Autodesk Fusion 360 part; units mm, degrees
(part 2 of 3)
sketch "Skizze15" plane through (0, 0, -33) normal (0, 0, -1) x (1, 0, 0)
  line L0 (-5.3, -15.5) -> (-3.8, -15.5)
  line L1 (-3.8, -15.5) -> (-3.8, -12.5)
  line L2 (-3.8, -12.5) -> (-2, -12.5)
  line L3 (-2, -12.5) -> (-2, -15.5)
  line L4 (-2, -15.5) -> (-0.5, -15.5)
  line L5 (-0.5, -15.5) -> (-0.5, 0.5)
  line L6 (-0.5, 0.5) -> (77.5, 0.5)
  line L7 (77.5, 0.5) -> (77.5, -50)
  line L8 (77.5, -50) -> (-0.5, -50)
  line L9 (-0.5, -50) -> (-0.5, -21.5)
  line L10 (-0.5, -21.5) -> (-2, -21.5)
  line L11 (-2, -21.5) -> (-2, -24.5)
  line L12 (-2, -24.5) -> (-3.8, -24.5)
  line L13 (-3.8, -24.5) -> (-3.8, -21.5)
  line L14 (-3.8, -21.5) -> (-5.3, -21.5)
  line L15 (-5.3, -21.5) -> (-5.3, -26)
  line L16 (-5.3, -26) -> (-2, -26)
  line L17 (-2, -26) -> (-2, -51.5)
  line L18 (-2, -51.5) -> (79, -51.5)
  line L19 (79, -51.5) -> (79, 2)
  line L20 (79, 2) -> (-2, 2)
  line L21 (-2, 2) -> (-2, -11)
  line L22 (-2, -11) -> (-5.3, -11)
  line L23 (-5.3, -11) -> (-5.3, -15.5)
  line L24 (-0.4, -21.4) -> (-2.1, -21.4)
  line L25 (-2.1, -21.4) -> (-2.1, -24.4)
  line L26 (-2.1, -24.4) -> (-3.7, -24.4)
  line L27 (-3.7, -24.4) -> (-3.7, -21.4)
  line L28 (-3.7, -21.4) -> (-5.4, -21.4)
  line L29 (-5.4, -21.4) -> (-5.4, -26.1)
  line L30 (-5.4, -26.1) -> (-2.1, -26.1)
  line L31 (-2.1, -26.1) -> (-2.1, -51.6)
  line L32 (-2.1, -51.6) -> (79.1, -51.6)
  line L33 (79.1, -51.6) -> (79.1, 2.1)
  line L34 (79.1, 2.1) -> (-2.1, 2.1)
  line L35 (-2.1, 2.1) -> (-2.1, -10.9)
  line L36 (-2.1, -10.9) -> (-5.4, -10.9)
  line L37 (-5.4, -10.9) -> (-5.4, -15.6)
  line L38 (-5.4, -15.6) -> (-3.7, -15.6)
  line L39 (-3.7, -15.6) -> (-3.7, -12.6)
  line L40 (-3.7, -12.6) -> (-2.1, -12.6)
  line L41 (-2.1, -12.6) -> (-2.1, -15.6)
  line L42 (-2.1, -15.6) -> (-0.4, -15.6)
  line L43 (-0.4, -15.6) -> (-0.4, 0.4)
  line L44 (-0.4, 0.4) -> (77.4, 0.4)
  line L45 (77.4, 0.4) -> (77.4, -49.9)
  line L46 (77.4, -49.9) -> (-0.4, -49.9)
  line L47 (-0.4, -49.9) -> (-0.4, -21.4)
  line L48 (-0.4, -21.4) -> (-0.4, -15.6)
  line L49 (-0.4, -49.9) -> (77.4, -49.9)
  line L50 (77.4, -49.9) -> (77.4, 0.4)
  line L51 (77.4, 0.4) -> (-0.4, 0.4)
  line L52 (-0.4, 0.4) -> (-0.4, -49.9)
  line L53 (75.9, -1.1) -> (1.1, -1.1)
  line L54 (1.1, -1.1) -> (1.1, -48.4)
  line L55 (1.1, -48.4) -> (75.9, -48.4)
  line L56 (75.9, -48.4) -> (75.9, -1.1)
  line L57 (-5.4, -21.4) -> (-5.4, -15.5)
  line L58 (-5.3, -21.5) -> (-5.3, -15.5)
  dimension "d73" = 0.1
  dimension "d74" = -1.5
  constraint horizontal L49
  constraint vertical L50
  constraint horizontal L51
  constraint vertical L52
  constraint coincident L37 L57.end
  constraint coincident L14.end L15.start
  constraint coincident L0.start L23.end
extrude "Extrusion20" add sketch "Skizze15" along normal blind 1.5 separate body contours L0 L1 L2 L3 L4 L5 L6 L7 L8 L9 L10 L11 L12 L13 L14 L15 L16 L17 L18 L19 L20 L21 L22 L23 | L0 L1 L2 L3 L4 L5 L6 L7 L8 L9 L10 L11 L12 L13 L14 L24 L25 L26 L27 L28 L38 L39 L40 L41 L42 L43 L44 L45 L46 L47 L49 L50 L51 L52 L58 | L24 L25 L26 L27 L28 L38 L39 L40 L41 L42 L48 L52 L58 | L43 L44 L45 L46 L47 L48 L49 L50 L51 L52 | L53 L54 L55 L56 makes body 4
sketch "Skizze16" plane through (0, 0, -34.5) normal (0, 0, -1) x (1, 0, 0)
  line L0 (-5.3, -26) -> (-2, -26)
  line L1 (-2, -26) -> (-2, -51.5)
  line L2 (-2, -51.5) -> (79, -51.5)
  line L3 (79, -51.5) -> (79, 2)
  line L4 (79, 2) -> (-2, 2)
  line L5 (-2, 2) -> (-2, -11)
  line L6 (-2, -11) -> (-5.3, -11)
  line L7 (-5.3, -11) -> (-5.3, -26)
  line L8 (1.1, -48.4) -> (75.9, -48.4)
  line L9 (75.9, -48.4) -> (75.9, -1.1)
  line L10 (75.9, -1.1) -> (1.1, -1.1)
  line L11 (1.1, -1.1) -> (1.1, -48.4)
  line L12 (1.1, -48.4) -> (75.9, -48.4)
  line L13 (-0.4, -49.9) -> (-0.4, 0.4)
  line L14 (-0.4, 0.4) -> (77.4, 0.4)
  line L15 (77.4, 0.4) -> (77.4, -49.9)
  line L16 (77.4, -49.9) -> (-0.4, -49.9)
  line L17 (-2, -51.5) -> (79, 2) construction
  line L18 (-2, 2) -> (79, -51.5) construction
  line L19 (53, -5.5) -> (24, -5.5)
  arc A0 (24, -5.5) -> (24, -44) centre (24, -24.75) ccw
  line L20 (24, -44) -> (53, -44)
  arc A1 (53, -44) -> (53, -5.5) centre (53, -24.75) ccw
  line L21 (53, -24.75) -> (24, -24.75) construction
  line L22 (-89.8785, -69.1132) -> (-94.8785, -66.2265)
  line L23 (-94.8785, -66.2265) -> (-99.8785, -69.1132)
  line L24 (-99.8785, -69.1132) -> (-99.8785, -74.8868)
  line L25 (-99.8785, -74.8868) -> (-94.8785, -77.7735)
  line L26 (-94.8785, -77.7735) -> (-89.8785, -74.8868)
  line L27 (-89.8785, -74.8868) -> (-89.8785, -69.1132)
  line L28 (-94.8785, -77.7735) -> (6, -77.7735)
  line L29 (-83.1871, -71.0235) -> (-78.1871, -68.1368)
  line L30 (-78.1871, -68.1368) -> (-78.1871, -62.3632)
  line L31 (-78.1871, -62.3632) -> (-83.1871, -59.4765)
  line L32 (-83.1871, -59.4765) -> (-88.1871, -62.3632)
  line L33 (-88.1871, -62.3632) -> (-88.1871, -68.1368)
  line L34 (-88.1871, -68.1368) -> (-83.1871, -71.0235)
  line L35 (-71.4958, -64.2735) -> (-66.4958, -61.3868)
  line L36 (-66.4958, -61.3868) -> (-66.4958, -55.6132)
  line L37 (-66.4958, -55.6132) -> (-71.4958, -52.7265)
  line L38 (-71.4958, -52.7265) -> (-76.4958, -55.6132)
  line L39 (-76.4958, -55.6132) -> (-76.4958, -61.3868)
  line L40 (-76.4958, -61.3868) -> (-71.4958, -64.2735)
  line L41 (-59.8044, -57.5235) -> (-54.8044, -54.6368)
  line L42 (-54.8044, -54.6368) -> (-54.8044, -48.8632)
  line L43 (-54.8044, -48.8632) -> (-59.8044, -45.9765)
  line L44 (-59.8044, -45.9765) -> (-64.8044, -48.8632)
  line L45 (-64.8044, -48.8632) -> (-64.8044, -54.6368)
  line L46 (-64.8044, -54.6368) -> (-59.8044, -57.5235)
  line L47 (-48.1131, -50.7735) -> (-43.1131, -47.8868)
  line L48 (-43.1131, -47.8868) -> (-43.1131, -42.1132)
  line L49 (-43.1131, -42.1132) -> (-48.1131, -39.2265)
  line L50 (-48.1131, -39.2265) -> (-53.1131, -42.1132)
  line L51 (-53.1131, -42.1132) -> (-53.1131, -47.8868)
  line L52 (-53.1131, -47.8868) -> (-48.1131, -50.7735)
  line L53 (-36.4217, -44.0235) -> (-31.4217, -41.1368)
  line L54 (-31.4217, -41.1368) -> (-31.4217, -35.3632)
  line L55 (-31.4217, -35.3632) -> (-36.4217, -32.4765)
  line L56 (-36.4217, -32.4765) -> (-41.4217, -35.3632)
  line L57 (-41.4217, -35.3632) -> (-41.4217, -41.1368)
  line L58 (-41.4217, -41.1368) -> (-36.4217, -44.0235)
  line L59 (-24.7304, -37.2735) -> (-19.7304, -34.3868)
  line L60 (-19.7304, -34.3868) -> (-19.7304, -28.6132)
  line L61 (-19.7304, -28.6132) -> (-24.7304, -25.7265)
  line L62 (-24.7304, -25.7265) -> (-29.7304, -28.6132)
  line L63 (-29.7304, -28.6132) -> (-29.7304, -34.3868)
  line L64 (-29.7304, -34.3868) -> (-24.7304, -37.2735)
  line L65 (-13.0391, -30.5235) -> (-8.0391, -27.6368)
  line L66 (-8.0391, -27.6368) -> (-8.0391, -21.8632)
  line L67 (-8.0391, -21.8632) -> (-13.0391, -18.9765)
  line L68 (-13.0391, -18.9765) -> (-18.0391, -21.8632)
  line L69 (-18.0391, -21.8632) -> (-18.0391, -27.6368)
  line L70 (-18.0391, -27.6368) -> (-13.0391, -30.5235)
  line L71 (-1.3477, -23.7735) -> (3.6523, -20.8868)
  line L72 (3.6523, -20.8868) -> (3.6523, -15.1132)
  line L73 (3.6523, -15.1132) -> (-1.3477, -12.2265)
  line L74 (-1.3477, -12.2265) -> (-6.3477, -15.1132)
  line L75 (-6.3477, -15.1132) -> (-6.3477, -20.8868)
  line L76 (-6.3477, -20.8868) -> (-1.3477, -23.7735)
  line L77 (10.3436, -17.0235) -> (15.3436, -14.1368)
  line L78 (15.3436, -14.1368) -> (15.3436, -8.3632)
  line L79 (15.3436, -8.3632) -> (10.3436, -5.4765)
  line L80 (10.3436, -5.4765) -> (5.3436, -8.3632)
  line L81 (5.3436, -8.3632) -> (5.3436, -14.1368)
  line L82 (5.3436, -14.1368) -> (10.3436, -17.0235)
  line L83 (22.035, -10.2735) -> (27.035, -7.3868)
  line L84 (27.035, -7.3868) -> (27.035, -1.6132)
  line L85 (27.035, -1.6132) -> (22.035, 1.2735)
  line L86 (22.035, 1.2735) -> (17.035, -1.6132)
  line L87 (17.035, -1.6132) -> (17.035, -7.3868)
  line L88 (17.035, -7.3868) -> (22.035, -10.2735)
  line L89 (-70.8785, -77.7735) -> (-65.8785, -74.8868)
  line L90 (-65.8785, -74.8868) -> (-65.8785, -69.1132)
  line L91 (-65.8785, -69.1132) -> (-70.8785, -66.2265)
  line L92 (-70.8785, -66.2265) -> (-75.8785, -69.1132)
  line L93 (-75.8785, -69.1132) -> (-75.8785, -74.8868)
  line L94 (-75.8785, -74.8868) -> (-70.8785, -77.7735)
  line L95 (-59.1871, -71.0235) -> (-54.1871, -68.1368)
  line L96 (-54.1871, -68.1368) -> (-54.1871, -62.3632)
  line L97 (-54.1871, -62.3632) -> (-59.1871, -59.4765)
  line L98 (-59.1871, -59.4765) -> (-64.1871, -62.3632)
  line L99 (-64.1871, -62.3632) -> (-64.1871, -68.1368)
  line L100 (-64.1871, -68.1368) -> (-59.1871, -71.0235)
  line L101 (-47.4958, -64.2735) -> (-42.4958, -61.3868)
  line L102 (-42.4958, -61.3868) -> (-42.4958, -55.6132)
  line L103 (-42.4958, -55.6132) -> (-47.4958, -52.7265)
  line L104 (-47.4958, -52.7265) -> (-52.4958, -55.6132)
  line L105 (-52.4958, -55.6132) -> (-52.4958, -61.3868)
  line L106 (-52.4958, -61.3868) -> (-47.4958, -64.2735)
  line L107 (-35.8044, -57.5235) -> (-30.8044, -54.6368)
  line L108 (-30.8044, -54.6368) -> (-30.8044, -48.8632)
  line L109 (-30.8044, -48.8632) -> (-35.8044, -45.9765)
  line L110 (-35.8044, -45.9765) -> (-40.8044, -48.8632)
  line L111 (-40.8044, -48.8632) -> (-40.8044, -54.6368)
  line L112 (-40.8044, -54.6368) -> (-35.8044, -57.5235)
  line L113 (-24.1131, -50.7735) -> (-19.1131, -47.8868)
  line L114 (-19.1131, -47.8868) -> (-19.1131, -42.1132)
  line L115 (-19.1131, -42.1132) -> (-24.1131, -39.2265)
  line L116 (-24.1131, -39.2265) -> (-29.1131, -42.1132)
  line L117 (-29.1131, -42.1132) -> (-29.1131, -47.8868)
  line L118 (-29.1131, -47.8868) -> (-24.1131, -50.7735)
  line L119 (-12.4217, -44.0235) -> (-7.4217, -41.1368)
  line L120 (-7.4217, -41.1368) -> (-7.4217, -35.3632)
  line L121 (-7.4217, -35.3632) -> (-12.4217, -32.4765)
  line L122 (-12.4217, -32.4765) -> (-17.4217, -35.3632)
  line L123 (-17.4217, -35.3632) -> (-17.4217, -41.1368)
  line L124 (-17.4217, -41.1368) -> (-12.4217, -44.0235)
  line L125 (-0.7304, -37.2735) -> (4.2696, -34.3868)
  line L126 (4.2696, -34.3868) -> (4.2696, -28.6132)
  line L127 (4.2696, -28.6132) -> (-0.7304, -25.7265)
  line L128 (-0.7304, -25.7265) -> (-5.7304, -28.6132)
  line L129 (-5.7304, -28.6132) -> (-5.7304, -34.3868)
  line L130 (-5.7304, -34.3868) -> (-0.7304, -37.2735)
  line L131 (10.9609, -30.5235) -> (15.9609, -27.6368)
  line L132 (15.9609, -27.6368) -> (15.9609, -21.8632)
  line L133 (15.9609, -21.8632) -> (10.9609, -18.9765)
  line L134 (10.9609, -18.9765) -> (5.9609, -21.8632)
  line L135 (5.9609, -21.8632) -> (5.9609, -27.6368)
  line L136 (5.9609, -27.6368) -> (10.9609, -30.5235)
  line L137 (22.6523, -23.7735) -> (27.6523, -20.8868)
  line L138 (27.6523, -20.8868) -> (27.6523, -15.1132)
  line L139 (27.6523, -15.1132) -> (22.6523, -12.2265)
  line L140 (22.6523, -12.2265) -> (17.6523, -15.1132)
  line L141 (17.6523, -15.1132) -> (17.6523, -20.8868)
  line L142 (17.6523, -20.8868) -> (22.6523, -23.7735)
  line L143 (34.3436, -17.0235) -> (39.3436, -14.1368)
  line L144 (39.3436, -14.1368) -> (39.3436, -8.3632)
  line L145 (39.3436, -8.3632) -> (34.3436, -5.4765)
  line L146 (34.3436, -5.4765) -> (29.3436, -8.3632)
  line L147 (29.3436, -8.3632) -> (29.3436, -14.1368)
  line L148 (29.3436, -14.1368) -> (34.3436, -17.0235)
  line L149 (46.035, -10.2735) -> (51.035, -7.3868)
  line L150 (51.035, -7.3868) -> (51.035, -1.6132)
  line L151 (51.035, -1.6132) -> (46.035, 1.2735)
  line L152 (46.035, 1.2735) -> (41.035, -1.6132)
  line L153 (41.035, -1.6132) -> (41.035, -7.3868)
  line L154 (41.035, -7.3868) -> (46.035, -10.2735)
  line L155 (-46.8785, -77.7735) -> (-41.8785, -74.8868)
  line L156 (-41.8785, -74.8868) -> (-41.8785, -69.1132)
  line L157 (-41.8785, -69.1132) -> (-46.8785, -66.2265)
  line L158 (-46.8785, -66.2265) -> (-51.8785, -69.1132)
  line L159 (-51.8785, -69.1132) -> (-51.8785, -74.8868)
  line L160 (-51.8785, -74.8868) -> (-46.8785, -77.7735)
  line L161 (-35.1871, -71.0235) -> (-30.1871, -68.1368)
  line L162 (-30.1871, -68.1368) -> (-30.1871, -62.3632)
  line L163 (-30.1871, -62.3632) -> (-35.1871, -59.4765)
  line L164 (-35.1871, -59.4765) -> (-40.1871, -62.3632)
  line L165 (-40.1871, -62.3632) -> (-40.1871, -68.1368)
  line L166 (-40.1871, -68.1368) -> (-35.1871, -71.0235)
  line L167 (-23.4958, -64.2735) -> (-18.4958, -61.3868)
  line L168 (-18.4958, -61.3868) -> (-18.4958, -55.6132)
  line L169 (-18.4958, -55.6132) -> (-23.4958, -52.7265)
  line L170 (-23.4958, -52.7265) -> (-28.4958, -55.6132)
  line L171 (-28.4958, -55.6132) -> (-28.4958, -61.3868)
  line L172 (-28.4958, -61.3868) -> (-23.4958, -64.2735)
  line L173 (-11.8044, -57.5235) -> (-6.8044, -54.6368)
  line L174 (-6.8044, -54.6368) -> (-6.8044, -48.8632)
  line L175 (-6.8044, -48.8632) -> (-11.8044, -45.9765)
  line L176 (-11.8044, -45.9765) -> (-16.8044, -48.8632)
  line L177 (-16.8044, -48.8632) -> (-16.8044, -54.6368)
  line L178 (-16.8044, -54.6368) -> (-11.8044, -57.5235)
  line L179 (-0.1131, -50.7735) -> (4.8869, -47.8868)
  line L180 (4.8869, -47.8868) -> (4.8869, -42.1132)
  line L181 (4.8869, -42.1132) -> (-0.1131, -39.2265)
  line L182 (-0.1131, -39.2265) -> (-5.1131, -42.1132)
  line L183 (-5.1131, -42.1132) -> (-5.1131, -47.8868)
  line L184 (-5.1131, -47.8868) -> (-0.1131, -50.7735)
  line L185 (11.5783, -44.0235) -> (16.5783, -41.1368)
  line L186 (16.5783, -41.1368) -> (16.5783, -35.3632)
  line L187 (16.5783, -35.3632) -> (11.5783, -32.4765)
  line L188 (11.5783, -32.4765) -> (6.5783, -35.3632)
  line L189 (6.5783, -35.3632) -> (6.5783, -41.1368)
  line L190 (6.5783, -41.1368) -> (11.5783, -44.0235)
  line L191 (23.2696, -37.2735) -> (28.2696, -34.3868)
  line L192 (28.2696, -34.3868) -> (28.2696, -28.6132)
  line L193 (28.2696, -28.6132) -> (23.2696, -25.7265)
  line L194 (23.2696, -25.7265) -> (18.2696, -28.6132)
  line L195 (18.2696, -28.6132) -> (18.2696, -34.3868)
  line L196 (18.2696, -34.3868) -> (23.2696, -37.2735)
  line L197 (34.9609, -30.5235) -> (39.9609, -27.6368)
  line L198 (39.9609, -27.6368) -> (39.9609, -21.8632)
  line L199 (39.9609, -21.8632) -> (34.9609, -18.9765)
  line L200 (34.9609, -18.9765) -> (29.9609, -21.8632)
  line L201 (29.9609, -21.8632) -> (29.9609, -27.6368)
  line L202 (29.9609, -27.6368) -> (34.9609, -30.5235)
  line L203 (46.6523, -23.7735) -> (51.6523, -20.8868)
  line L204 (51.6523, -20.8868) -> (51.6523, -15.1132)
  line L205 (51.6523, -15.1132) -> (46.6523, -12.2265)
  line L206 (46.6523, -12.2265) -> (41.6523, -15.1132)
  line L207 (41.6523, -15.1132) -> (41.6523, -20.8868)
  line L208 (41.6523, -20.8868) -> (46.6523, -23.7735)
  line L209 (58.3436, -17.0235) -> (63.3436, -14.1368)
  line L210 (63.3436, -14.1368) -> (63.3436, -8.3632)
  line L211 (63.3436, -8.3632) -> (58.3436, -5.4765)
  line L212 (58.3436, -5.4765) -> (53.3436, -8.3632)
  line L213 (53.3436, -8.3632) -> (53.3436, -14.1368)
  line L214 (53.3436, -14.1368) -> (58.3436, -17.0235)
  line L215 (70.035, -10.2735) -> (75.035, -7.3868)
  line L216 (75.035, -7.3868) -> (75.035, -1.6132)
  line L217 (75.035, -1.6132) -> (70.035, 1.2735)
  line L218 (70.035, 1.2735) -> (65.035, -1.6132)
  line L219 (65.035, -1.6132) -> (65.035, -7.3868)
  line L220 (65.035, -7.3868) -> (70.035, -10.2735)
  line L221 (-22.8785, -77.7735) -> (-17.8785, -74.8868)
  line L222 (-17.8785, -74.8868) -> (-17.8785, -69.1132)
  line L223 (-17.8785, -69.1132) -> (-22.8785, -66.2265)
  line L224 (-22.8785, -66.2265) -> (-27.8785, -69.1132)
  line L225 (-27.8785, -69.1132) -> (-27.8785, -74.8868)
  line L226 (-27.8785, -74.8868) -> (-22.8785, -77.7735)
  line L227 (-11.1871, -71.0235) -> (-6.1871, -68.1368)
  line L228 (-6.1871, -68.1368) -> (-6.1871, -62.3632)
  line L229 (-6.1871, -62.3632) -> (-11.1871, -59.4765)
  line L230 (-11.1871, -59.4765) -> (-16.1871, -62.3632)
  line L231 (-16.1871, -62.3632) -> (-16.1871, -68.1368)
  line L232 (-16.1871, -68.1368) -> (-11.1871, -71.0235)
  line L233 (0.5042, -64.2735) -> (5.5042, -61.3868)
  line L234 (5.5042, -61.3868) -> (5.5042, -55.6132)
  line L235 (5.5042, -55.6132) -> (0.5042, -52.7265)
  line L236 (0.5042, -52.7265) -> (-4.4958, -55.6132)
  line L237 (-4.4958, -55.6132) -> (-4.4958, -61.3868)
  line L238 (-4.4958, -61.3868) -> (0.5042, -64.2735)
  line L239 (12.1956, -57.5235) -> (17.1956, -54.6368)
  line L240 (17.1956, -54.6368) -> (17.1956, -48.8632)
  line L241 (17.1956, -48.8632) -> (12.1956, -45.9765)
  line L242 (12.1956, -45.9765) -> (7.1956, -48.8632)
  line L243 (7.1956, -48.8632) -> (7.1956, -54.6368)
  line L244 (7.1956, -54.6368) -> (12.1956, -57.5235)
  line L245 (23.8869, -50.7735) -> (28.8869, -47.8868)
  line L246 (28.8869, -47.8868) -> (28.8869, -42.1132)
  line L247 (28.8869, -42.1132) -> (23.8869, -39.2265)
  line L248 (23.8869, -39.2265) -> (18.8869, -42.1132)
  line L249 (18.8869, -42.1132) -> (18.8869, -47.8868)
  line L250 (18.8869, -47.8868) -> (23.8869, -50.7735)
  line L251 (35.5783, -44.0235) -> (40.5783, -41.1368)
  line L252 (40.5783, -41.1368) -> (40.5783, -35.3632)
  line L253 (40.5783, -35.3632) -> (35.5783, -32.4765)
  line L254 (35.5783, -32.4765) -> (30.5783, -35.3632)
  line L255 (30.5783, -35.3632) -> (30.5783, -41.1368)
  line L256 (30.5783, -41.1368) -> (35.5783, -44.0235)
  line L257 (47.2696, -37.2735) -> (52.2696, -34.3868)
  line L258 (52.2696, -34.3868) -> (52.2696, -28.6132)
  line L259 (52.2696, -28.6132) -> (47.2696, -25.7265)
  line L260 (47.2696, -25.7265) -> (42.2696, -28.6132)
  line L261 (42.2696, -28.6132) -> (42.2696, -34.3868)
  line L262 (42.2696, -34.3868) -> (47.2696, -37.2735)
  line L263 (58.9609, -30.5235) -> (63.9609, -27.6368)
  line L264 (63.9609, -27.6368) -> (63.9609, -21.8632)
  line L265 (63.9609, -21.8632) -> (58.9609, -18.9765)
  line L266 (58.9609, -18.9765) -> (53.9609, -21.8632)
  line L267 (53.9609, -21.8632) -> (53.9609, -27.6368)
  line L268 (53.9609, -27.6368) -> (58.9609, -30.5235)
  line L269 (70.6523, -23.7735) -> (75.6523, -20.8868)
  line L270 (75.6523, -20.8868) -> (75.6523, -15.1132)
  line L271 (75.6523, -15.1132) -> (70.6523, -12.2265)
  line L272 (70.6523, -12.2265) -> (65.6523, -15.1132)
  line L273 (65.6523, -15.1132) -> (65.6523, -20.8868)
  line L274 (65.6523, -20.8868) -> (70.6523, -23.7735)
  line L275 (82.3436, -17.0235) -> (87.3436, -14.1368)
  line L276 (87.3436, -14.1368) -> (87.3436, -8.3632)
  line L277 (87.3436, -8.3632) -> (82.3436, -5.4765)
  line L278 (82.3436, -5.4765) -> (77.3436, -8.3632)
  line L279 (77.3436, -8.3632) -> (77.3436, -14.1368)
  line L280 (77.3436, -14.1368) -> (82.3436, -17.0235)
  line L281 (94.035, -10.2735) -> (99.035, -7.3868)
  line L282 (99.035, -7.3868) -> (99.035, -1.6132)
  line L283 (99.035, -1.6132) -> (94.035, 1.2735)
  line L284 (94.035, 1.2735) -> (89.035, -1.6132)
  line L285 (89.035, -1.6132) -> (89.035, -7.3868)
  line L286 (89.035, -7.3868) -> (94.035, -10.2735)
  line L287 (1.1215, -77.7735) -> (6.1215, -74.8868)
  line L288 (6.1215, -74.8868) -> (6.1215, -69.1132)
  line L289 (6.1215, -69.1132) -> (1.1215, -66.2265)
  line L290 (1.1215, -66.2265) -> (-3.8785, -69.1132)
  line L291 (-3.8785, -69.1132) -> (-3.8785, -74.8868)
  line L292 (-3.8785, -74.8868) -> (1.1215, -77.7735)
  line L293 (12.8129, -71.0235) -> (17.8129, -68.1368)
  line L294 (17.8129, -68.1368) -> (17.8129, -62.3632)
  line L295 (17.8129, -62.3632) -> (12.8129, -59.4765)
  line L296 (12.8129, -59.4765) -> (7.8129, -62.3632)
  line L297 (7.8129, -62.3632) -> (7.8129, -68.1368)
  line L298 (7.8129, -68.1368) -> (12.8129, -71.0235)
  line L299 (24.5042, -64.2735) -> (29.5042, -61.3868)
  line L300 (29.5042, -61.3868) -> (29.5042, -55.6132)
  line L301 (29.5042, -55.6132) -> (24.5042, -52.7265)
  line L302 (24.5042, -52.7265) -> (19.5042, -55.6132)
  line L303 (19.5042, -55.6132) -> (19.5042, -61.3868)
  line L304 (19.5042, -61.3868) -> (24.5042, -64.2735)
  line L305 (36.1956, -57.5235) -> (41.1956, -54.6368)
  line L306 (41.1956, -54.6368) -> (41.1956, -48.8632)
  line L307 (41.1956, -48.8632) -> (36.1956, -45.9765)
  line L308 (36.1956, -45.9765) -> (31.1956, -48.8632)
  line L309 (31.1956, -48.8632) -> (31.1956, -54.6368)
  line L310 (31.1956, -54.6368) -> (36.1956, -57.5235)
  line L311 (47.8869, -50.7735) -> (52.8869, -47.8868)
  line L312 (52.8869, -47.8868) -> (52.8869, -42.1132)
  line L313 (52.8869, -42.1132) -> (47.8869, -39.2265)
  line L314 (47.8869, -39.2265) -> (42.8869, -42.1132)
  line L315 (42.8869, -42.1132) -> (42.8869, -47.8868)
  line L316 (42.8869, -47.8868) -> (47.8869, -50.7735)
  line L317 (59.5783, -44.0235) -> (64.5783, -41.1368)
  line L318 (64.5783, -41.1368) -> (64.5783, -35.3632)
  line L319 (64.5783, -35.3632) -> (59.5783, -32.4765)
  line L320 (59.5783, -32.4765) -> (54.5783, -35.3632)
  line L321 (54.5783, -35.3632) -> (54.5783, -41.1368)
  line L322 (54.5783, -41.1368) -> (59.5783, -44.0235)
  line L323 (71.2696, -37.2735) -> (76.2696, -34.3868)
  line L324 (76.2696, -34.3868) -> (76.2696, -28.6132)
  line L325 (76.2696, -28.6132) -> (71.2696, -25.7265)
  line L326 (71.2696, -25.7265) -> (66.2696, -28.6132)
  line L327 (66.2696, -28.6132) -> (66.2696, -34.3868)
  line L328 (66.2696, -34.3868) -> (71.2696, -37.2735)
  line L329 (82.9609, -30.5235) -> (87.9609, -27.6368)
  line L330 (87.9609, -27.6368) -> (87.9609, -21.8632)
  line L331 (87.9609, -21.8632) -> (82.9609, -18.9765)
  line L332 (82.9609, -18.9765) -> (77.9609, -21.8632)
  line L333 (77.9609, -21.8632) -> (77.9609, -27.6368)
  line L334 (77.9609, -27.6368) -> (82.9609, -30.5235)
  line L335 (94.6523, -23.7735) -> (99.6523, -20.8868)
  line L336 (99.6523, -20.8868) -> (99.6523, -15.1132)
  line L337 (99.6523, -15.1132) -> (94.6523, -12.2265)
  line L338 (94.6523, -12.2265) -> (89.6523, -15.1132)
  line L339 (89.6523, -15.1132) -> (89.6523, -20.8868)
  line L340 (89.6523, -20.8868) -> (94.6523, -23.7735)
  line L341 (106.3436, -17.0235) -> (111.3436, -14.1368)
  line L342 (111.3436, -14.1368) -> (111.3436, -8.3632)
  line L343 (111.3436, -8.3632) -> (106.3436, -5.4765)
  line L344 (106.3436, -5.4765) -> (101.3436, -8.3632)
  line L345 (101.3436, -8.3632) -> (101.3436, -14.1368)
  line L346 (101.3436, -14.1368) -> (106.3436, -17.0235)
  line L347 (118.035, -10.2735) -> (123.035, -7.3868)
  line L348 (123.035, -7.3868) -> (123.035, -1.6132)
  line L349 (123.035, -1.6132) -> (118.035, 1.2735)
  line L350 (118.035, 1.2735) -> (113.035, -1.6132)
  line L351 (113.035, -1.6132) -> (113.035, -7.3868)
  line L352 (113.035, -7.3868) -> (118.035, -10.2735)
  line L353 (25.1215, -77.7735) -> (30.1215, -74.8868)
  line L354 (30.1215, -74.8868) -> (30.1215, -69.1132)
  line L355 (30.1215, -69.1132) -> (25.1215, -66.2265)
  line L356 (25.1215, -66.2265) -> (20.1215, -69.1132)
  line L357 (20.1215, -69.1132) -> (20.1215, -74.8868)
  line L358 (20.1215, -74.8868) -> (25.1215, -77.7735)
  line L359 (36.8129, -71.0235) -> (41.8129, -68.1368)
  line L360 (41.8129, -68.1368) -> (41.8129, -62.3632)
  line L361 (41.8129, -62.3632) -> (36.8129, -59.4765)
  line L362 (36.8129, -59.4765) -> (31.8129, -62.3632)
  line L363 (31.8129, -62.3632) -> (31.8129, -68.1368)
  line L364 (31.8129, -68.1368) -> (36.8129, -71.0235)
  line L365 (48.5042, -64.2735) -> (53.5042, -61.3868)
  line L366 (53.5042, -61.3868) -> (53.5042, -55.6132)
  line L367 (53.5042, -55.6132) -> (48.5042, -52.7265)
  line L368 (48.5042, -52.7265) -> (43.5042, -55.6132)
  line L369 (43.5042, -55.6132) -> (43.5042, -61.3868)
  line L370 (43.5042, -61.3868) -> (48.5042, -64.2735)
  line L371 (60.1956, -57.5235) -> (65.1956, -54.6368)
  line L372 (65.1956, -54.6368) -> (65.1956, -48.8632)
  line L373 (65.1956, -48.8632) -> (60.1956, -45.9765)
  line L374 (60.1956, -45.9765) -> (55.1956, -48.8632)
  line L375 (55.1956, -48.8632) -> (55.1956, -54.6368)
  line L376 (55.1956, -54.6368) -> (60.1956, -57.5235)
  line L377 (71.8869, -50.7735) -> (76.8869, -47.8868)
  line L378 (76.8869, -47.8868) -> (76.8869, -42.1132)
  line L379 (76.8869, -42.1132) -> (71.8869, -39.2265)
  line L380 (71.8869, -39.2265) -> (66.8869, -42.1132)
  line L381 (66.8869, -42.1132) -> (66.8869, -47.8868)
  line L382 (66.8869, -47.8868) -> (71.8869, -50.7735)
  line L383 (83.5783, -44.0235) -> (88.5783, -41.1368)
  line L384 (88.5783, -41.1368) -> (88.5783, -35.3632)
  line L385 (88.5783, -35.3632) -> (83.5783, -32.4765)
  line L386 (83.5783, -32.4765) -> (78.5783, -35.3632)
  line L387 (78.5783, -35.3632) -> (78.5783, -41.1368)
  line L388 (78.5783, -41.1368) -> (83.5783, -44.0235)
  line L389 (95.2696, -37.2735) -> (100.2696, -34.3868)
  line L390 (100.2696, -34.3868) -> (100.2696, -28.6132)
  line L391 (100.2696, -28.6132) -> (95.2696, -25.7265)
  line L392 (95.2696, -25.7265) -> (90.2696, -28.6132)
  line L393 (90.2696, -28.6132) -> (90.2696, -34.3868)
  line L394 (90.2696, -34.3868) -> (95.2696, -37.2735)
  line L395 (106.9609, -30.5235) -> (111.9609, -27.6368)
  line L396 (111.9609, -27.6368) -> (111.9609, -21.8632)
  line L397 (111.9609, -21.8632) -> (106.9609, -18.9765)
  line L398 (106.9609, -18.9765) -> (101.9609, -21.8632)
  line L399 (101.9609, -21.8632) -> (101.9609, -27.6368)
  line L400 (101.9609, -27.6368) -> (106.9609, -30.5235)
  line L401 (118.6523, -23.7735) -> (123.6523, -20.8868)
  line L402 (123.6523, -20.8868) -> (123.6523, -15.1132)
  line L403 (123.6523, -15.1132) -> (118.6523, -12.2265)
  line L404 (118.6523, -12.2265) -> (113.6523, -15.1132)
  line L405 (113.6523, -15.1132) -> (113.6523, -20.8868)
  line L406 (113.6523, -20.8868) -> (118.6523, -23.7735)
  line L407 (130.3436, -17.0235) -> (135.3436, -14.1368)
  line L408 (135.3436, -14.1368) -> (135.3436, -8.3632)
  line L409 (135.3436, -8.3632) -> (130.3436, -5.4765)
  line L410 (130.3436, -5.4765) -> (125.3436, -8.3632)
  line L411 (125.3436, -8.3632) -> (125.3436, -14.1368)
  line L412 (125.3436, -14.1368) -> (130.3436, -17.0235)
  line L413 (142.035, -10.2735) -> (147.035, -7.3868)
  line L414 (147.035, -7.3868) -> (147.035, -1.6132)
  line L415 (147.035, -1.6132) -> (142.035, 1.2735)
  line L416 (142.035, 1.2735) -> (137.035, -1.6132)
  line L417 (137.035, -1.6132) -> (137.035, -7.3868)
  line L418 (137.035, -7.3868) -> (142.035, -10.2735)
  line L419 (49.1215, -77.7735) -> (54.1215, -74.8868)
  line L420 (54.1215, -74.8868) -> (54.1215, -69.1132)
  line L421 (54.1215, -69.1132) -> (49.1215, -66.2265)
  line L422 (49.1215, -66.2265) -> (44.1215, -69.1132)
  line L423 (44.1215, -69.1132) -> (44.1215, -74.8868)
  line L424 (44.1215, -74.8868) -> (49.1215, -77.7735)
  line L425 (60.8129, -71.0235) -> (65.8129, -68.1368)
  line L426 (65.8129, -68.1368) -> (65.8129, -62.3632)
  line L427 (65.8129, -62.3632) -> (60.8129, -59.4765)
  line L428 (60.8129, -59.4765) -> (55.8129, -62.3632)
  line L429 (55.8129, -62.3632) -> (55.8129, -68.1368)
  line L430 (55.8129, -68.1368) -> (60.8129, -71.0235)
  line L431 (72.5042, -64.2735) -> (77.5042, -61.3868)
  line L432 (77.5042, -61.3868) -> (77.5042, -55.6132)
  line L433 (77.5042, -55.6132) -> (72.5042, -52.7265)
  line L434 (72.5042, -52.7265) -> (67.5042, -55.6132)
  line L435 (67.5042, -55.6132) -> (67.5042, -61.3868)
  line L436 (67.5042, -61.3868) -> (72.5042, -64.2735)
  line L437 (84.1956, -57.5235) -> (89.1956, -54.6368)
  line L438 (89.1956, -54.6368) -> (89.1956, -48.8632)
  line L439 (89.1956, -48.8632) -> (84.1956, -45.9765)
  line L440 (84.1956, -45.9765) -> (79.1956, -48.8632)
  line L441 (79.1956, -48.8632) -> (79.1956, -54.6368)
  line L442 (79.1956, -54.6368) -> (84.1956, -57.5235)
  line L443 (95.8869, -50.7735) -> (100.8869, -47.8868)
  line L444 (100.8869, -47.8868) -> (100.8869, -42.1132)
  line L445 (100.8869, -42.1132) -> (95.8869, -39.2265)
  line L446 (95.8869, -39.2265) -> (90.8869, -42.1132)
  line L447 (90.8869, -42.1132) -> (90.8869, -47.8868)
  line L448 (90.8869, -47.8868) -> (95.8869, -50.7735)
  line L449 (107.5783, -44.0235) -> (112.5783, -41.1368)
  line L450 (112.5783, -41.1368) -> (112.5783, -35.3632)
  line L451 (112.5783, -35.3632) -> (107.5783, -32.4765)
  line L452 (107.5783, -32.4765) -> (102.5783, -35.3632)
  line L453 (102.5783, -35.3632) -> (102.5783, -41.1368)
  line L454 (102.5783, -41.1368) -> (107.5783, -44.0235)
  line L455 (119.2696, -37.2735) -> (124.2696, -34.3868)
  line L456 (124.2696, -34.3868) -> (124.2696, -28.6132)
  line L457 (124.2696, -28.6132) -> (119.2696, -25.7265)
  line L458 (119.2696, -25.7265) -> (114.2696, -28.6132)
  line L459 (114.2696, -28.6132) -> (114.2696, -34.3868)
  line L460 (114.2696, -34.3868) -> (119.2696, -37.2735)
  line L461 (130.9609, -30.5235) -> (135.9609, -27.6368)
  line L462 (135.9609, -27.6368) -> (135.9609, -21.8632)
  line L463 (135.9609, -21.8632) -> (130.9609, -18.9765)
  line L464 (130.9609, -18.9765) -> (125.9609, -21.8632)
  line L465 (125.9609, -21.8632) -> (125.9609, -27.6368)
  line L466 (125.9609, -27.6368) -> (130.9609, -30.5235)
  line L467 (142.6523, -23.7735) -> (147.6523, -20.8868)
  line L468 (147.6523, -20.8868) -> (147.6523, -15.1132)
  line L469 (147.6523, -15.1132) -> (142.6523, -12.2265)
  line L470 (142.6523, -12.2265) -> (137.6523, -15.1132)
  line L471 (137.6523, -15.1132) -> (137.6523, -20.8868)
  line L472 (137.6523, -20.8868) -> (142.6523, -23.7735)
  line L473 (154.3436, -17.0235) -> (159.3436, -14.1368)
  line L474 (159.3436, -14.1368) -> (159.3436, -8.3632)
  line L475 (159.3436, -8.3632) -> (154.3436, -5.4765)
  line L476 (154.3436, -5.4765) -> (149.3436, -8.3632)
  line L477 (149.3436, -8.3632) -> (149.3436, -14.1368)
  line L478 (149.3436, -14.1368) -> (154.3436, -17.0235)
  line L479 (166.035, -10.2735) -> (171.035, -7.3868)
  line L480 (171.035, -7.3868) -> (171.035, -1.6132)
  line L481 (171.035, -1.6132) -> (166.035, 1.2735)
  line L482 (166.035, 1.2735) -> (161.035, -1.6132)
  line L483 (161.035, -1.6132) -> (161.035, -7.3868)
  line L484 (161.035, -7.3868) -> (166.035, -10.2735)
  line L485 (73.1215, -77.7735) -> (78.1215, -74.8868)
  line L486 (78.1215, -74.8868) -> (78.1215, -69.1132)
  line L487 (78.1215, -69.1132) -> (73.1215, -66.2265)
  line L488 (73.1215, -66.2265) -> (68.1215, -69.1132)
  line L489 (68.1215, -69.1132) -> (68.1215, -74.8868)
  line L490 (68.1215, -74.8868) -> (73.1215, -77.7735)
  line L491 (84.8129, -71.0235) -> (89.8129, -68.1368)
  line L492 (89.8129, -68.1368) -> (89.8129, -62.3632)
  line L493 (89.8129, -62.3632) -> (84.8129, -59.4765)
  line L494 (84.8129, -59.4765) -> (79.8129, -62.3632)
  line L495 (79.8129, -62.3632) -> (79.8129, -68.1368)
  line L496 (79.8129, -68.1368) -> (84.8129, -71.0235)
  line L497 (96.5042, -64.2735) -> (101.5042, -61.3868)
  line L498 (101.5042, -61.3868) -> (101.5042, -55.6132)
  line L499 (101.5042, -55.6132) -> (96.5042, -52.7265)
  line L500 (96.5042, -52.7265) -> (91.5042, -55.6132)
  line L501 (91.5042, -55.6132) -> (91.5042, -61.3868)
  line L502 (91.5042, -61.3868) -> (96.5042, -64.2735)
  line L503 (108.1956, -57.5235) -> (113.1956, -54.6368)
  line L504 (113.1956, -54.6368) -> (113.1956, -48.8632)
  line L505 (113.1956, -48.8632) -> (108.1956, -45.9765)
  line L506 (108.1956, -45.9765) -> (103.1956, -48.8632)
  line L507 (103.1956, -48.8632) -> (103.1956, -54.6368)
  line L508 (103.1956, -54.6368) -> (108.1956, -57.5235)
  line L509 (119.8869, -50.7735) -> (124.8869, -47.8868)
  line L510 (124.8869, -47.8868) -> (124.8869, -42.1132)
  line L511 (124.8869, -42.1132) -> (119.8869, -39.2265)
  line L512 (119.8869, -39.2265) -> (114.8869, -42.1132)
  line L513 (114.8869, -42.1132) -> (114.8869, -47.8868)
  line L514 (114.8869, -47.8868) -> (119.8869, -50.7735)
  line L515 (131.5783, -44.0235) -> (136.5783, -41.1368)
  line L516 (136.5783, -41.1368) -> (136.5783, -35.3632)
  line L517 (136.5783, -35.3632) -> (131.5783, -32.4765)
  line L518 (131.5783, -32.4765) -> (126.5783, -35.3632)
  line L519 (126.5783, -35.3632) -> (126.5783, -41.1368)
  line L520 (126.5783, -41.1368) -> (131.5783, -44.0235)
  line L521 (143.2696, -37.2735) -> (148.2696, -34.3868)
  line L522 (148.2696, -34.3868) -> (148.2696, -28.6132)
  line L523 (148.2696, -28.6132) -> (143.2696, -25.7265)
  line L524 (143.2696, -25.7265) -> (138.2696, -28.6132)
  line L525 (138.2696, -28.6132) -> (138.2696, -34.3868)
  line L526 (138.2696, -34.3868) -> (143.2696, -37.2735)
  line L527 (154.9609, -30.5235) -> (159.9609, -27.6368)
  line L528 (159.9609, -27.6368) -> (159.9609, -21.8632)
  line L529 (159.9609, -21.8632) -> (154.9609, -18.9765)
  line L530 (154.9609, -18.9765) -> (149.9609, -21.8632)
  line L531 (149.9609, -21.8632) -> (149.9609, -27.6368)
  line L532 (149.9609, -27.6368) -> (154.9609, -30.5235)
  line L533 (166.6523, -23.7735) -> (171.6523, -20.8868)
  line L534 (171.6523, -20.8868) -> (171.6523, -15.1132)
  line L535 (171.6523, -15.1132) -> (166.6523, -12.2265)
  line L536 (166.6523, -12.2265) -> (161.6523, -15.1132)
  line L537 (161.6523, -15.1132) -> (161.6523, -20.8868)
  line L538 (161.6523, -20.8868) -> (166.6523, -23.7735)
  line L539 (178.3436, -17.0235) -> (183.3436, -14.1368)
  line L540 (183.3436, -14.1368) -> (183.3436, -8.3632)
  line L541 (183.3436, -8.3632) -> (178.3436, -5.4765)
  line L542 (178.3436, -5.4765) -> (173.3436, -8.3632)
  line L543 (173.3436, -8.3632) -> (173.3436, -14.1368)
  line L544 (173.3436, -14.1368) -> (178.3436, -17.0235)
  line L545 (190.035, -10.2735) -> (195.035, -7.3868)
  line L546 (195.035, -7.3868) -> (195.035, -1.6132)
  line L547 (195.035, -1.6132) -> (190.035, 1.2735)
  line L548 (190.035, 1.2735) -> (185.035, -1.6132)
  line L549 (185.035, -1.6132) -> (185.035, -7.3868)
  line L550 (185.035, -7.3868) -> (190.035, -10.2735)
  line L551 (97.1215, -77.7735) -> (102.1215, -74.8868)
  line L552 (102.1215, -74.8868) -> (102.1215, -69.1132)
  line L553 (102.1215, -69.1132) -> (97.1215, -66.2265)
  line L554 (97.1215, -66.2265) -> (92.1215, -69.1132)
  line L555 (92.1215, -69.1132) -> (92.1215, -74.8868)
  line L556 (92.1215, -74.8868) -> (97.1215, -77.7735)
  line L557 (108.8129, -71.0235) -> (113.8129, -68.1368)
  line L558 (113.8129, -68.1368) -> (113.8129, -62.3632)
  line L559 (113.8129, -62.3632) -> (108.8129, -59.4765)
  line L560 (108.8129, -59.4765) -> (103.8129, -62.3632)
  line L561 (103.8129, -62.3632) -> (103.8129, -68.1368)
  line L562 (103.8129, -68.1368) -> (108.8129, -71.0235)
  line L563 (120.5042, -64.2735) -> (125.5042, -61.3868)
  line L564 (125.5042, -61.3868) -> (125.5042, -55.6132)
  line L565 (125.5042, -55.6132) -> (120.5042, -52.7265)
  line L566 (120.5042, -52.7265) -> (115.5042, -55.6132)
  line L567 (115.5042, -55.6132) -> (115.5042, -61.3868)
  line L568 (115.5042, -61.3868) -> (120.5042, -64.2735)
  line L569 (132.1956, -57.5235) -> (137.1956, -54.6368)
  line L570 (137.1956, -54.6368) -> (137.1956, -48.8632)
  line L571 (137.1956, -48.8632) -> (132.1956, -45.9765)
  line L572 (132.1956, -45.9765) -> (127.1956, -48.8632)
  line L573 (127.1956, -48.8632) -> (127.1956, -54.6368)
  line L574 (127.1956, -54.6368) -> (132.1956, -57.5235)
  line L575 (143.8869, -50.7735) -> (148.8869, -47.8868)
  line L576 (148.8869, -47.8868) -> (148.8869, -42.1132)
  line L577 (148.8869, -42.1132) -> (143.8869, -39.2265)
  line L578 (143.8869, -39.2265) -> (138.8869, -42.1132)
  line L579 (138.8869, -42.1132) -> (138.8869, -47.8868)
  line L580 (138.8869, -47.8868) -> (143.8869, -50.7735)
  line L581 (155.5783, -44.0235) -> (160.5783, -41.1368)
  line L582 (160.5783, -41.1368) -> (160.5783, -35.3632)
  line L583 (160.5783, -35.3632) -> (155.5783, -32.4765)
  line L584 (155.5783, -32.4765) -> (150.5783, -35.3632)
  line L585 (150.5783, -35.3632) -> (150.5783, -41.1368)
  line L586 (150.5783, -41.1368) -> (155.5783, -44.0235)
  line L587 (167.2696, -37.2735) -> (172.2696, -34.3868)
  line L588 (172.2696, -34.3868) -> (172.2696, -28.6132)
  line L589 (172.2696, -28.6132) -> (167.2696, -25.7265)
  line L590 (167.2696, -25.7265) -> (162.2696, -28.6132)
  line L591 (162.2696, -28.6132) -> (162.2696, -34.3868)
  line L592 (162.2696, -34.3868) -> (167.2696, -37.2735)
  line L593 (178.9609, -30.5235) -> (183.9609, -27.6368)
  line L594 (183.9609, -27.6368) -> (183.9609, -21.8632)
  line L595 (183.9609, -21.8632) -> (178.9609, -18.9765)
  line L596 (178.9609, -18.9765) -> (173.9609, -21.8632)
  line L597 (173.9609, -21.8632) -> (173.9609, -27.6368)
  line L598 (173.9609, -27.6368) -> (178.9609, -30.5235)
  line L599 (190.6523, -23.7735) -> (195.6523, -20.8868)
  line L600 (195.6523, -20.8868) -> (195.6523, -15.1132)
  line L601 (195.6523, -15.1132) -> (190.6523, -12.2265)
  line L602 (190.6523, -12.2265) -> (185.6523, -15.1132)
  line L603 (185.6523, -15.1132) -> (185.6523, -20.8868)
  line L604 (185.6523, -20.8868) -> (190.6523, -23.7735)
  line L605 (202.3436, -17.0235) -> (207.3436, -14.1368)
  line L606 (207.3436, -14.1368) -> (207.3436, -8.3632)
  line L607 (207.3436, -8.3632) -> (202.3436, -5.4765)
  line L608 (202.3436, -5.4765) -> (197.3436, -8.3632)
  line L609 (197.3436, -8.3632) -> (197.3436, -14.1368)
  line L610 (197.3436, -14.1368) -> (202.3436, -17.0235)
  line L611 (214.035, -10.2735) -> (219.035, -7.3868)
  line L612 (219.035, -7.3868) -> (219.035, -1.6132)
  line L613 (219.035, -1.6132) -> (214.035, 1.2735)
  line L614 (214.035, 1.2735) -> (209.035, -1.6132)
  line L615 (209.035, -1.6132) -> (209.035, -7.3868)
  line L616 (209.035, -7.3868) -> (214.035, -10.2735)
  point P0 (38.5, -24.75)
  point P1 (-94.8785, -72)
  dimension "d79" = 5
  dimension "d82" = 135
  dimension "d83" = 192
  constraint coincident L1.end L2.start
  constraint coincident L3.end L4.start
  constraint coincident L4.end L5.start
  constraint coincident L2.end L3.start
  constraint tangent L19 A0
  constraint tangent A0 L20
  constraint parallel L19 L20
  constraint tangent L20 A1
  constraint tangent L19 A1
  constraint horizontal L21
  constraint midpoint L18 P0
  constraint midpoint L21 P0
  constraint horizontal L28
  measures "d79" distance of P1 L27
extrude "Extrusion22" cut sketch "Skizze16" against normal blind 7 contours L19 A0 L83 L84 L87 L88 | A0 L77 L78 L79 L82 | L19 L149 L150 L153 L154 | L19 L143 L144 L145 L146 L147 L148 | A0 L185 L186 L187 L188 | A0 L20 L246 L247 L248 L249 | A1 L325 L326 L327 L328 | A1 L209 L210 L212 L213 L214 | L20 L312 L313 L314 L315 | L20 L251 L252 L253 L254 L255 L256 | A1 L269 L272 L273 L274 | A1 L318 L319 L320 L321 L322 | L131 L132 L133 L134 L135 L136 | L137 L138 L139 L140 L141 L142 | L191 L192 L193 L194 L195 L196 | L197 L198 L199 L200 L201 L202 | L203 L204 L205 L206 L207 L208 | L257 L258 L259 L260 L261 L262 | L263 L264 L265 L266 L267 L268 bodies 4
sketch "Skizze17" plane through (0, 51.5, 0) normal (0, 1, 0) x (-1, 0, 0)
  line L0 (-46.5552, -15.5) -> (-46.5552, -20.5)
  line L1 (-46.5552, -20.5) -> (-50.8853, -23)
  line L2 (-50.8853, -23) -> (-55.2155, -20.5)
  line L3 (-55.2155, -20.5) -> (-55.2155, -15.5)
  line L4 (-55.2155, -15.5) -> (-50.8853, -13)
  line L5 (-50.8853, -13) -> (-46.5552, -15.5)
  line L6 (-17.5384, -29.7827) -> (-26.1986, -29.7827)
  line L7 (-26.1986, -29.7827) -> (-26.1986, -26.25)
  line L8 (-26.1986, -26.25) -> (-21.8685, -23.75)
  line L9 (-21.8685, -23.75) -> (-17.5384, -26.25)
  line L10 (-17.5384, -26.25) -> (-17.5384, -29.7827)
  line L11 (-39.8447, -4.75) -> (-39.8447, -9.75)
  line L12 (-39.8447, -9.75) -> (-44.1749, -12.25)
  line L13 (-44.1749, -12.25) -> (-48.505, -9.75)
  line L14 (-48.505, -9.75) -> (-48.505, -4.75)
  line L15 (-48.505, -4.75) -> (-46.5591, -3.6265)
  line L16 (-46.5591, -3.6265) -> (-41.7907, -3.6265)
  line L17 (-41.7907, -3.6265) -> (-39.8447, -4.75)
  arc A0 (-4.1925, -22.4552) -> (-3.3748, -13.0727) centre (-15.9385, -16.7046) ccw
  line L18 (-4.1925, -22.4552) -> (-7.5791, -20.5)
  line L19 (-7.5791, -20.5) -> (-7.5791, -15.5)
  line L20 (-7.5791, -15.5) -> (-3.3748, -13.0727)
  arc A1 (-4.6691, -10.0685) -> (-11.9249, -4.2576) centre (-15.9385, -16.7046) ccw
  line L21 (-4.6691, -10.0685) -> (-8.4476, -12.25)
  line L22 (-8.4476, -12.25) -> (-12.7777, -9.75)
  line L23 (-12.7777, -9.75) -> (-12.7777, -4.75)
  line L24 (-12.7777, -4.75) -> (-11.9249, -4.2576)
  line L25 (-16.0266, -4.75) -> (-16.0266, -9.75)
  line L26 (-16.0266, -9.75) -> (-20.3567, -12.25)
  line L27 (-20.3567, -12.25) -> (-24.6868, -9.75)
  line L28 (-24.6868, -9.75) -> (-24.6868, -4.75)
  line L29 (-24.6868, -4.75) -> (-22.7409, -3.6265)
  line L30 (-22.7409, -3.6265) -> (-17.9725, -3.6265)
  line L31 (-17.9725, -3.6265) -> (-16.0266, -4.75)
  line L32 (-51.7538, -4.75) -> (-51.7538, -9.75)
  line L33 (-51.7538, -9.75) -> (-56.084, -12.25)
  line L34 (-56.084, -12.25) -> (-60.4141, -9.75)
  line L35 (-60.4141, -9.75) -> (-60.4141, -6.7446)
  arc A2 (-53.5312, -3.7238) -> (-60.4141, -6.7446) centre (-51.9385, -16.7046) ccw
  line L36 (-53.5312, -3.7238) -> (-51.7538, -4.75)
  line L37 (-34.6461, -15.5) -> (-34.6461, -20.5)
  line L38 (-34.6461, -20.5) -> (-38.9762, -23)
  line L39 (-38.9762, -23) -> (-43.3064, -20.5)
  line L40 (-43.3064, -20.5) -> (-43.3064, -15.5)
  line L41 (-43.3064, -15.5) -> (-38.9762, -13)
  line L42 (-38.9762, -13) -> (-34.6461, -15.5)
  arc A3 (-61.2677, -25.87) -> (-53.2657, -29.7152) centre (-51.9385, -16.7046) ccw
  line L43 (-61.2677, -25.87) -> (-57.5958, -23.75)
  line L44 (-57.5958, -23.75) -> (-53.2657, -26.25)
  line L45 (-53.2657, -26.25) -> (-53.2657, -29.7152)
  line L46 (-29.4475, -29.7827) -> (-38.1077, -29.7827)
  line L47 (-38.1077, -29.7827) -> (-38.1077, -26.25)
  line L48 (-38.1077, -26.25) -> (-33.7776, -23.75)
  line L49 (-33.7776, -23.75) -> (-29.4475, -26.25)
  line L50 (-29.4475, -26.25) -> (-29.4475, -29.7827)
  line L51 (-27.9357, -4.75) -> (-27.9357, -9.75)
  line L52 (-27.9357, -9.75) -> (-32.2658, -12.25)
  line L53 (-32.2658, -12.25) -> (-36.5959, -9.75)
  line L54 (-36.5959, -9.75) -> (-36.5959, -4.75)
  line L55 (-36.5959, -4.75) -> (-34.65, -3.6265)
  line L56 (-34.65, -3.6265) -> (-29.8816, -3.6265)
  line L57 (-29.8816, -3.6265) -> (-27.9357, -4.75)
  arc A4 (-14.2896, -29.6784) -> (-6.4938, -25.7509) centre (-15.9385, -16.7046) ccw
  line L58 (-14.2896, -29.6784) -> (-14.2896, -26.25)
  line L59 (-14.2896, -26.25) -> (-9.9594, -23.75)
  line L60 (-9.9594, -23.75) -> (-6.4938, -25.7509)
  line L61 (-10.8279, -15.5) -> (-10.8279, -20.5)
  line L62 (-10.8279, -20.5) -> (-15.1581, -23)
  line L63 (-15.1581, -23) -> (-19.4882, -20.5)
  line L64 (-19.4882, -20.5) -> (-19.4882, -15.5)
  line L65 (-19.4882, -15.5) -> (-15.1581, -13)
  line L66 (-15.1581, -13) -> (-10.8279, -15.5)
  line L67 (-41.3566, -29.7827) -> (-50.0168, -29.7827)
  line L68 (-50.0168, -29.7827) -> (-50.0168, -26.25)
  line L69 (-50.0168, -26.25) -> (-45.6867, -23.75)
  line L70 (-45.6867, -23.75) -> (-41.3566, -26.25)
  line L71 (-41.3566, -26.25) -> (-41.3566, -29.7827)
  line L72 (-58.4643, -15.5) -> (-58.4643, -20.5)
  line L73 (-58.4643, -20.5) -> (-62.7944, -23)
  line L74 (-62.7944, -23) -> (-63.6632, -22.4984)
  arc A5 (-64.7619, -14.1359) -> (-63.6632, -22.4984) centre (-51.9385, -16.7046) ccw
  line L75 (-64.7619, -14.1359) -> (-62.7944, -13)
  line L76 (-62.7944, -13) -> (-58.4643, -15.5)
  line L77 (-22.737, -15.5) -> (-22.737, -20.5)
  line L78 (-22.737, -20.5) -> (-27.0672, -23)
  line L79 (-27.0672, -23) -> (-31.3973, -20.5)
  line L80 (-31.3973, -20.5) -> (-31.3973, -15.5)
  line L81 (-31.3973, -15.5) -> (-27.0672, -13)
  line L82 (-27.0672, -13) -> (-22.737, -15.5)
  line L83 (-71.5, -16) -> (-71.5, -20)
  line L84 (-71.5, -20) -> (-77.5, -20)
  line L85 (-77.5, -20) -> (-77.5, -16)
  line L86 (-77.5, -16) -> (-71.5, -16)
  line L87 (-79, 2) -> (-79, -33)
  line L88 (-79, -33) -> (2, -33)
  line L89 (2, -33) -> (2, 2)
  line L90 (2, 2) -> (-79, 2)
  line L91 (-77.5, -16) -> (-71.5, -16)
  line L92 (-71.5, -20) -> (-77.5, -20)
  line L93 (-77.5, -20) -> (-77.5, -16)
  line L94 (-71.65, -19.85) -> (-77.35, -19.85)
  line L95 (-77.35, -19.85) -> (-77.35, -16.15)
  line L96 (-77.35, -16.15) -> (-71.65, -16.15)
  line L97 (-71.65, -16.15) -> (-71.65, -19.85)
  line L98 (-78.5, -15) -> (-70.5, -15)
  line L99 (-70.5, -15) -> (-70.5, -21)
  line L100 (-70.5, -21) -> (-78.5, -21)
  line L101 (-78.5, -21) -> (-78.5, -15)
  dimension "d86" = 0.15
  dimension "d87" = -1
extrude "Extrusion23" add sketch "Skizze17" along normal blind 1.5 from surface at 0.2 separate body contours L83 L84 L85 L86 L91 L92 L93 | L94 L95 L96 L97 | L98 L99 L100 L101 makes body 5
extrude "Extrusion24" add sketch "Skizze17" along normal blind -12.5 and the other way blind -1 contours L94 L95 L96 L97 bodies 5
fillet "Abrundung1" radius 1.5 4 edges at (78.5, 52.45, -21) (78.5, 52.45, -15) (70.5, 52.45, -15) (70.5, 52.45, -21) on bodies 5
chamfer "Fase3" distance 1 angle 45 16 edges at (79, 51.5, -15.5) (79, -2, -15.5) (-2, 51.5, -15.5) (-2, -2, -15.5) (-5.3, 26, -15.5) (-2, 26, -15.5) (-2, 11, -15.5) (-5.3, 11, -15.5) (79, 51.5, -33.75) (79, -2, -33.75) (-2, 51.5, -33.75) (-2, -2, -33.75) (-5.3, 26, -33.75) (-2, 26, -33.75) (-2, 11, -33.75) (-5.3, 11, -33.75) on bodies 2 4
chamfer "Fase4" distance 1 angle 45 16 edges at (-2, 38.75, 2) (-2.5, 26.5, 2) (-3.65, 26, 2) (-4.8, 25.5, 2) (-5.3, 18.5, 2) (-4.8, 11.5, 2) (-3.65, 11, 2) (-2.5, 10.5, 2) (-2, 4.5, 2) (-1.5, -1.5, 2) (38.5, -2, 2) (78.5, -1.5, 2) (79, 24.75, 2) (78.5, 51, 2) (38.5, 51.5, 2) (-1.5, 51, 2) on bodies 2
chamfer "Fase5" distance 0.5 angle 45 17 edges at (-3.6, 24.3, -18.3) (79, 24.75, -34.5) (78.5, -1.5, -34.5) (38.5, -2, -34.5) (78.5, 51, -34.5) (38.5, 51.5, -34.5) (-1.5, 51, -34.5) (-2, 38.75, -34.5) (-2.5, 26.5, -34.5) (-4.8, 25.5, -34.5) (-3.65, 26, -34.5) (-5.3, 18.5, -34.5) (-4.8, 11.5, -34.5) (-3.65, 11, -34.5) (-2.5, 10.5, -34.5) (-2, 4.5, -34.5) (-1.5, -1.5, -34.5) on bodies 3 4
sketch "Skizze18" plane through (0, 0, -33) normal (0, 0, -1) x (1, 0, 0)
  line L0 (-5.3, -12) -> (-5.3, -15.5)
  line L1 (-5.3, -15.5) -> (-3.8, -15.5)
  line L2 (-3.8, -15.5) -> (-3.8, -12.5)
  line L3 (-3.8, -12.5) -> (-2, -12.5)
  line L4 (-2, -12.5) -> (-2, -15.5)
  line L5 (-2, -15.5) -> (-0.5, -15.5)
  line L6 (-0.5, -15.5) -> (-0.5, 0.5)
  line L7 (-0.5, 0.5) -> (77.5, 0.5)
  line L8 (77.5, 0.5) -> (77.5, -50)
  line L9 (77.5, -50) -> (-0.5, -50)
  line L10 (-0.5, -50) -> (-0.5, -21.5)
  line L11 (-0.5, -21.5) -> (-2, -21.5)
  line L12 (-2, -21.5) -> (-2, -24.5)
  line L13 (-2, -24.5) -> (-3.8, -24.5)
  line L14 (-3.8, -24.5) -> (-3.8, -21.5)
  line L15 (-3.8, -21.5) -> (-5.3, -21.5)
  line L16 (-5.3, -21.5) -> (-5.3, -25)
  line L17 (-4.3, -26) -> (-3, -26)
  line L18 (-1, -51.5) -> (78, -51.5)
  line L19 (79, -50.5) -> (79, 1)
  line L20 (78, 2) -> (-1, 2)
  line L21 (-3, -11) -> (-4.3, -11)
  line L22 (-0.5, 0.5) -> (2.5, 0.5)
  line L23 (2.5, 0.5) -> (2.5, -4.5)
  line L24 (2.5, -4.5) -> (-0.5, -4.5)
  line L25 (-0.5, -4.5) -> (-0.5, 0.5)
  line L26 (-0.5, -50) -> (2.5, -50)
  line L27 (2.5, -50) -> (2.5, -45)
  line L28 (2.5, -45) -> (-0.5, -45)
  line L29 (-0.5, -45) -> (-0.5, -50)
  line L30 (-4.3, -11) -> (-5.3, -12)
  line L31 (-5.3, -25) -> (-4.3, -26)
  line L32 (-3, -26) -> (-2, -27)
  line L33 (-2, -27) -> (-2, -50.5)
  line L34 (-2, -50.5) -> (-1, -51.5)
  line L35 (78, -51.5) -> (79, -50.5)
  line L36 (79, 1) -> (78, 2)
  line L37 (-1, 2) -> (-2, 1)
  line L38 (-2, 1) -> (-2, -10)
  line L39 (-2, -10) -> (-3, -11)
  dimension "d101" = 3
  dimension "d102" = 5
  dimension "d103" = 3
  dimension "d104" = 5
  constraint horizontal L22
  constraint vertical L23
  constraint horizontal L24
  constraint vertical L25
  constraint coincident L6.end L7.start
  constraint horizontal L26
  constraint vertical L27
  constraint horizontal L28
  constraint vertical L29
  constraint coincident L9.end L10.start
  measures "d101" distance of L6.end L22.end
  measures "d102" distance of L6.end L24.end
  measures "d103" distance of L9.end L26.end
  measures "d104" distance of L9.end L28.end
extrude "Extrusion25" add sketch "Skizze18" against normal blind 2 contours L6 L7 L22 L23 L24 L25 | L9 L10 L26 L27 L28 L29 bodies 2
sketch "Skizze19" plane through (0, 0, -33) normal (0, 0, -1) x (1, 0, 0)
  line L0 (-5.3, -12) -> (-5.3, -15.5)
  line L1 (-5.3, -15.5) -> (-3.8, -15.5)
  line L2 (-3.8, -15.5) -> (-3.8, -12.5)
  line L3 (-3.8, -12.5) -> (-2, -12.5)
  line L4 (-2, -12.5) -> (-2, -15.5)
  line L5 (-2, -15.5) -> (-0.5, -15.5)
  line L6 (-0.5, -15.5) -> (-0.5, -4.5)
  line L7 (-0.5, -4.5) -> (2.5, -4.5)
  line L8 (2.5, -4.5) -> (2.5, 0.5)
  line L9 (2.5, 0.5) -> (77.5, 0.5)
  line L10 (77.5, 0.5) -> (77.5, -50)
  line L11 (77.5, -50) -> (2.5, -50)
  line L12 (2.5, -50) -> (2.5, -45)
  line L13 (2.5, -45) -> (-0.5, -45)
  line L14 (-0.5, -45) -> (-0.5, -21.5)
  line L15 (-0.5, -21.5) -> (-2, -21.5)
  line L16 (-2, -21.5) -> (-2, -24.5)
  line L17 (-2, -24.5) -> (-3.8, -24.5)
  line L18 (-3.8, -24.5) -> (-3.8, -21.5)
  line L19 (-3.8, -21.5) -> (-5.3, -21.5)
  line L20 (-5.3, -21.5) -> (-5.3, -25)
  line L21 (-4.3, -26) -> (-3, -26)
  line L22 (-1, -51.5) -> (78, -51.5)
  line L23 (79, -50.5) -> (79, 1)
  line L24 (78, 2) -> (-1, 2)
  line L25 (-3, -11) -> (-4.3, -11)
  line L26 (-0.5, -4) -> (2, -4)
  line L27 (2, -4) -> (2, 0.5)
  line L28 (2, -50) -> (2, -45.5)
  line L29 (2, -45.5) -> (-0.5, -45.5)
  line L30 (2, 0.5) -> (-0.5, 0.5)
  line L31 (-0.5, 0.5) -> (-0.5, -4)
  line L32 (-0.5, -4) -> (2, -4)
  line L33 (2, -4) -> (2, 0.5)
  line L34 (-0.5, -45.5) -> (2, -45.5)
  line L35 (2, -45.5) -> (2, -50)
  line L36 (2, -50) -> (-0.5, -50)
  line L37 (-0.5, -50) -> (-0.5, -45.5)
  line L38 (-4.3, -11) -> (-5.3, -12)
  line L39 (-5.3, -25) -> (-4.3, -26)
  line L40 (-3, -26) -> (-2, -27)
  line L41 (-2, -27) -> (-2, -50.5)
  line L42 (-2, -50.5) -> (-1, -51.5)
  line L43 (78, -51.5) -> (79, -50.5)
  line L44 (79, 1) -> (78, 2)
  line L45 (-1, 2) -> (-2, 1)
  line L46 (-2, 1) -> (-2, -10)
  line L47 (-2, -10) -> (-3, -11)
  dimension "d107" = -0.5
  dimension "d108" = -0.5
  constraint horizontal L30
  constraint vertical L31
  constraint horizontal L32
  constraint vertical L33
  constraint horizontal L34
  constraint vertical L35
  constraint horizontal L36
  constraint vertical L37